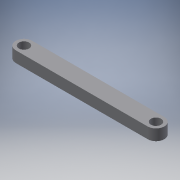
# Autodesk Inventor part: HbFingerMainCouplerLink01
Saved by Autodesk Inventor 2017 (Build 210142000, 142)
## iProperties
Created: 2015-02-23
Part Number: HbFingerMainCouplerLink01
Material: 一般
Document SubType Name: Modeling
Designer: Yamaura
Density: 1 g/cm^3
Appearance: 既定
Author: Yamaura
Autodesk Inventor part; units mm, degrees
ref_plane "YZ Plane" through (0, 0, 0) normal (1, 0, 0) x (0, 1, 0)
ref_plane "XZ Plane" through (0, 0, 0) normal (0, 1, 0) x (-1, 0, 0)
ref_plane "XY Plane" through (0, 0, 0) normal (0, 0, 1) x (1, 0, 0)
sketch "スケッチ1" plane through (0, 0, 0) normal (0, 0, 1) x (1, 0, 0)
  circle A0 centre (0, 0) radius 1.7
  circle A1 centre (48, 0) radius 1.7
  circle A2 centre (0, 0) radius 3
  circle A3 centre (48, 0) radius 3
  line L0 (0, 3) -> (48, 3)
  line L1 (0, -3) -> (48, -3)
  dimension "d0" = 3.4
  dimension "d1" = 3.4
  dimension "d2" = 6
  dimension "d3" = 6
  dimension "d4" = 48
  constraints: 4 centre point, 4 end point, 4 point on circle, 4 tangent, 3 coincident, 1 horizontal alignment
  measures "d0" diameter of A0
  measures "d1" diameter of A1
  measures "d2" diameter of A2
  measures "d3" diameter of A3
  measures "d4" distance of A1.centre point (0, 0)
extrude "押し出し1" add sketch "スケッチ1" along normal mid plane 4
offset faces "サイズ1" outward -0.05 faces at (49.6945, -0.1368, 0.6667)
offset faces "サイズ2" outward -0.05 faces at (1.6945, 0.1368, -0.6667)
scale "尺度1" factors (0.8836555, 0.8836555, 0.8836555) then translate (2.7923, 0.349, -0.2327) bodies 1
sketch "スケッチ2" plane through (2.7923, -2.3019, 1.5346) normal (0, 0, 1) x (1, 0, 0)
  circle A0 centre (0, 2.651) radius 1.5464 projected
  circle A1 centre (0, 2.651) radius 1.65
  circle A2 centre (42.4155, 2.651) radius 1.5464 projected
  circle A3 centre (42.4155, 2.651) radius 1.65
  point P0 (-2.7923, 2.3019)
  dimension "d12" = 3.3
  constraints: 2 centre point, 2 coincident, 1 equal radius
  measures "d12" diameter of A1
extrude "押し出し2" cut sketch "スケッチ2" against normal up to next
